Autodesk Inventor part; units mm, degrees
(part 3 of 3)
sketch "Sketch19" plane through (0, 0, -25.4) normal (0, 0, -1) x (-1, 0, 0)
  circle A0 centre (0, 0) radius 236.22 projected
  arc A1 (202.9027, -10.9875) -> (-203.2, 0) centre (0, 0) ccw construction
  circle A2 centre (0, 0) radius 127 construction
  line L0 (127.9212, -89.6882) -> (127.759, -89.2068)
  spline S0 degree 2 poles (127.759, -89.2068) (129.2741, -86.0586) (132.1163, -79.2182) knots 0 0 0 1 1 1
  spline S1 degree 2 poles (132.1163, -79.2182) (135.0319, -72.2013) (136.1206, -69.0829) knots 0 0 0 1 1 1
  line L1 (136.1206, -69.0829) -> (136.5138, -68.884)
  line L2 (136.5138, -68.884) -> (138.7645, -69.8192)
  line L3 (138.7645, -69.8192) -> (138.945, -70.2565)
  spline S2 degree 2 poles (138.945, -70.2565) (137.728, -73.6838) (137.6586, -74.2243) knots 0 0 0 1 1 1
  spline S3 degree 2 poles (137.6586, -74.2243) (137.52, -75.3052) (138.4359, -75.841) knots 0 0 0 1 1 1
  spline S4 degree 2 poles (138.4359, -75.841) (140.5915, -77.2542) (148.4027, -80.4998) knots 0 0 0 1 1 1
  line L4 (148.4027, -80.4998) -> (170.5125, -89.6866)
  line L5 (170.5125, -89.6866) -> (158.5776, -76.1887)
  spline S5 degree 2 poles (158.5776, -76.1887) (157.5986, -75.0575) (151.177, -68.0939) knots 0 0 0 1 1 1
  line L6 (151.177, -68.0939) -> (140.5896, -56.7084)
  line L7 (140.5896, -56.7084) -> (141.5064, -54.5019)
  spline S6 degree 2 poles (141.5064, -54.5019) (146.2817, -54.4678) (153.6703, -54.1223) knots 0 0 0 1 1 1
  line L8 (153.6703, -54.1223) -> (165.2679, -53.6109)
  line L9 (165.2679, -53.6109) -> (186.6543, -52.4575)
  line L10 (186.6543, -52.4575) -> (163.9708, -43.0323)
  spline S7 degree 2 poles (163.9708, -43.0323) (156.1596, -39.7867) (153.6556, -39.212) knots 0 0 0 1 1 1
  spline S8 degree 2 poles (153.6556, -39.212) (152.6113, -38.9851) (151.9615, -39.8019) knots 0 0 0 1 1 1
  spline S9 degree 2 poles (151.9615, -39.8019) (151.6274, -40.2323) (150.0572, -43.5129) knots 0 0 0 1 1 1
  line L11 (150.0572, -43.5129) -> (149.62, -43.6935)
  line L12 (149.62, -43.6935) -> (147.3693, -42.7583)
  line L13 (147.3693, -42.7583) -> (147.2328, -42.3394)
  spline S10 degree 2 poles (147.2328, -42.3394) (148.968, -38.6616) (150.3249, -35.3958) knots 0 0 0 1 1 1
  spline S11 degree 2 poles (150.3249, -35.3958) (151.8836, -31.6447) (153.284, -27.776) knots 0 0 0 1 1 1
  line L14 (153.284, -27.776) -> (153.6772, -27.5771)
  line L15 (153.6772, -27.5771) -> (155.9279, -28.5123)
  line L16 (155.9279, -28.5123) -> (156.1084, -28.9496)
  spline S12 degree 2 poles (156.1084, -28.9496) (154.8913, -32.3769) (154.822, -32.9174) knots 0 0 0 1 1 1
  spline S13 degree 2 poles (154.822, -32.9174) (154.7017, -33.9542) (155.5993, -34.5341) knots 0 0 0 1 1 1
  spline S14 degree 2 poles (155.5993, -34.5341) (157.7549, -35.9473) (165.5661, -39.1929) knots 0 0 0 1 1 1
  line L17 (165.5661, -39.1929) -> (182.8656, -46.381)
  spline S15 degree 2 poles (182.8656, -46.381) (190.6327, -49.6083) (193.1991, -50.1572) knots 0 0 0 1 1 1
  spline S16 degree 2 poles (193.1991, -50.1572) (194.1993, -50.3657) (194.8491, -49.549) knots 0 0 0 1 1 1
  spline S17 degree 2 poles (194.8491, -49.549) (195.1832, -49.1186) (196.7533, -45.8379) knots 0 0 0 1 1 1
  line L18 (196.7533, -45.8379) -> (197.2348, -45.6757)
  line L19 (197.2348, -45.6757) -> (199.4413, -46.5926)
  line L20 (199.4413, -46.5926) -> (199.6219, -47.0298)
  spline S18 degree 2 poles (199.6219, -47.0298) (197.9893, -50.3363) (195.8255, -55.5438) knots 0 0 0 1 1 1
  spline S19 degree 2 poles (195.8255, -55.5438) (194.1569, -59.5597) (193.1489, -62.6082) knots 0 0 0 1 1 1
  spline S20 degree 2 poles (193.1489, -62.6082) (190.2192, -62.6846) (184.8485, -62.7818) knots 0 0 0 1 1 1
  line L21 (184.8485, -62.7818) -> (179.4852, -62.9856)
  line L22 (179.4852, -62.9856) -> (153.401, -64.3605)
  line L23 (153.401, -64.3605) -> (161.4791, -73.5648)
  line L24 (161.4791, -73.5648) -> (174.9592, -88.3257)
  spline S21 degree 2 poles (174.9592, -88.3257) (177.3293, -90.9665) (180.2397, -93.6766) knots 0 0 0 1 1 1
  spline S22 degree 2 poles (180.2397, -93.6766) (178.4788, -97.292) (177.947, -98.5718) knots 0 0 0 1 1 1
  spline S23 degree 2 poles (177.947, -98.5718) (175.2881, -104.9708) (174.0969, -108.4606) knots 0 0 0 1 1 1
  line L25 (174.0969, -108.4606) -> (173.6412, -108.6853)
  line L26 (173.6412, -108.6853) -> (171.3905, -107.7501)
  line L27 (171.3905, -107.7501) -> (171.2283, -107.2687)
  spline S24 degree 2 poles (171.2283, -107.2687) (172.4271, -103.8855) (172.4964, -103.345) knots 0 0 0 1 1 1
  spline S25 degree 2 poles (172.4964, -103.345) (172.635, -102.2641) (171.7816, -101.7025) knots 0 0 0 1 1 1
  spline S26 degree 2 poles (171.7816, -101.7025) (169.5635, -100.3152) (161.7964, -97.0879) knots 0 0 0 1 1 1
  line L28 (161.7964, -97.0879) -> (144.497, -89.8998)
  spline S27 degree 2 poles (144.497, -89.8998) (136.6857, -86.6541) (134.1817, -86.0795) knots 0 0 0 1 1 1
  spline S28 degree 2 poles (134.1817, -86.0795) (133.1375, -85.8526) (132.4693, -86.7134) knots 0 0 0 1 1 1
  spline S29 degree 2 poles (132.4693, -86.7134) (132.1352, -87.1439) (130.5834, -90.3804) knots 0 0 0 1 1 1
  line L29 (130.5834, -90.3804) -> (130.1278, -90.6051)
  line L30 (130.1278, -90.6051) -> (127.9212, -89.6882)
  line L31 (96.1488, -143.05) -> (96.1692, -142.5097)
  spline S30 degree 2 poles (96.1692, -142.5097) (97.389, -140.6622) (96.6476, -138.808) (92.3916, -134.2169) knots 0 0 0 1 2 2 2
  spline S31 degree 2 poles (92.3916, -134.2169) (90.3448, -132.0089) (88.1527, -130.066) knots 0 0 0 1 1 1
  spline S32 degree 2 poles (88.1527, -130.066) (93.7904, -118.7143) (100.8699, -112.1516) knots 0 0 0 1 1 1
  spline S33 degree 2 poles (100.8699, -112.1516) (110.1574, -103.5421) (131.3344, -103.3298) (139.6516, -112.3018) knots 0 0 0 1 2 2 2
  spline S34 degree 2 poles (139.6516, -112.3018) (150.5028, -124.0075) (144.9851, -138.441) knots 0 0 0 1 1 1
  spline S35 degree 2 poles (144.9851, -138.441) (142.4707, -145.0075) (135.286, -151.6677) knots 0 0 0 1 1 1
  spline S36 degree 2 poles (135.286, -151.6677) (131.1505, -155.5014) (126.03, -158.5538) knots 0 0 0 1 1 1
  spline S37 degree 2 poles (126.03, -158.5538) (121.8106, -161.0317) (118.9006, -161.9698) knots 0 0 0 1 1 1
  line L32 (118.9006, -161.9698) -> (118.268, -161.7091)
  spline S38 degree 2 poles (118.268, -161.7091) (116.7896, -158.7787) (111.9795, -152.7463) knots 0 0 0 1 1 1
  line L33 (111.9795, -152.7463) -> (112.035, -152.1735)
  line L34 (112.035, -152.1735) -> (113.5771, -150.744)
  line L35 (113.5771, -150.744) -> (114.0823, -150.7969)
  spline S39 degree 2 poles (114.0823, -150.7969) (114.5372, -151.2876) (117.6065, -154.1768) (118.3665, -154.6452) knots 0 0 0 1 2 2 2
  spline S40 degree 2 poles (118.3665, -154.6452) (120.9175, -155.1476) (124.7259, -153.7025) knots 0 0 0 1 1 1
  spline S41 degree 2 poles (124.7259, -153.7025) (128.7095, -152.095) (132.1441, -148.911) knots 0 0 0 1 1 1
  spline S42 degree 2 poles (132.1441, -148.911) (141.3614, -140.3665) (137.9785, -129.6877) knots 0 0 0 1 1 1
  spline S43 degree 2 poles (137.9785, -129.6877) (136.4068, -124.7586) (132.2157, -120.2375) knots 0 0 0 1 1 1
  spline S44 degree 2 poles (132.2157, -120.2375) (125.523, -113.0178) (117.2819, -111.8602) knots 0 0 0 1 1 1
  spline S45 degree 2 poles (117.2819, -111.8602) (108.7056, -110.6223) (102.292, -116.5678) knots 0 0 0 1 1 1
  spline S46 degree 2 poles (102.292, -116.5678) (98.8924, -119.7192) (97.0352, -124.1126) knots 0 0 0 1 1 1
  spline S47 degree 2 poles (97.0352, -124.1126) (98.5494, -126.0975) (101.5058, -129.2868) knots 0 0 0 1 1 1
  spline S48 degree 2 poles (101.5058, -129.2868) (103.8775, -131.8452) (104.5726, -132.2435) knots 0 0 0 1 1 1
  spline S49 degree 2 poles (104.5726, -132.2435) (105.1052, -132.4666) (106.1062, -131.9296) knots 0 0 0 1 1 1
  spline S50 degree 2 poles (106.1062, -131.9296) (106.9371, -131.42) (110.8795, -128.2215) knots 0 0 0 1 1 1
  line L36 (110.8795, -128.2215) -> (111.3873, -128.207)
  line L37 (111.3873, -128.207) -> (112.9143, -129.8542)
  line L38 (112.9143, -129.8542) -> (112.8613, -130.3594)
  spline S51 degree 2 poles (112.8613, -130.3594) (108.9788, -133.7631) (104.8757, -137.6318) knots 0 0 0 1 1 1
  spline S52 degree 2 poles (104.8757, -137.6318) (102.525, -139.8761) (97.8262, -144.2971) knots 0 0 0 1 1 1
  line L39 (97.8262, -144.2971) -> (97.3184, -144.3117)
  line L40 (97.3184, -144.3117) -> (96.1488, -143.05)
  line L41 (26.9755, -152.7156) -> (27.1725, -152.2854)
  spline S53 degree 2 poles (27.1725, -152.2854) (30.5538, -151.2323) (37.4968, -148.651) knots 0 0 0 1 1 1
  spline S54 degree 2 poles (37.4968, -148.651) (44.5743, -146.0198) (47.6432, -144.6749) knots 0 0 0 1 1 1
  line L42 (47.6432, -144.6749) -> (48.0567, -144.8271)
  line L43 (48.0567, -144.8271) -> (48.906, -147.1115)
  line L44 (48.906, -147.1115) -> (48.6642, -147.5583)
  spline S55 degree 2 poles (48.6642, -147.5583) (45.3713, -148.9865) (44.8837, -149.3207) knots 0 0 0 1 1 1
  spline S56 degree 2 poles (44.8837, -149.3207) (44.043, -149.9392) (44.2302, -150.9913) knots 0 0 0 1 1 1
  spline S57 degree 2 poles (44.2302, -150.9913) (44.7097, -153.5152) (47.6573, -161.4437) knots 0 0 0 1 1 1
  line L45 (47.6573, -161.4437) -> (50.6216, -169.417)
  spline S58 degree 2 poles (50.6216, -169.417) (52.3456, -168.98) (61.4387, -165.5994) knots 0 0 0 1 1 1
  spline S59 degree 2 poles (61.4387, -165.5994) (69.8152, -162.4852) (72.3914, -161.3235) knots 0 0 0 1 1 1
  line L46 (72.3914, -161.3235) -> (69.4271, -153.3502)
  spline S60 degree 2 poles (69.4271, -153.3502) (66.4794, -145.4217) (65.1489, -143.2142) knots 0 0 0 1 1 1
  spline S61 degree 2 poles (65.1489, -143.2142) (64.6481, -142.2787) (63.5627, -142.3763) knots 0 0 0 1 1 1
  spline S62 degree 2 poles (63.5627, -142.3763) (63.02, -142.4251) (59.5491, -143.5116) knots 0 0 0 1 1 1
  line L47 (59.5491, -143.5116) -> (59.119, -143.3146)
  line L48 (59.119, -143.3146) -> (58.2863, -141.0749)
  line L49 (58.2863, -141.0749) -> (58.4833, -140.6448)
  spline S63 degree 2 poles (58.4833, -140.6448) (61.8646, -139.5916) (68.7629, -137.027) knots 0 0 0 1 1 1
  spline S64 degree 2 poles (68.7629, -137.027) (75.8851, -134.3791) (78.9093, -133.0508) knots 0 0 0 1 1 1
  line L50 (78.9093, -133.0508) -> (79.3675, -133.1864)
  line L51 (79.3675, -133.1864) -> (80.2168, -135.4709)
  line L52 (80.2168, -135.4709) -> (79.9751, -135.9176)
  spline S65 degree 2 poles (79.9751, -135.9176) (76.6821, -137.3458) (76.1946, -137.68) knots 0 0 0 1 1 1
  spline S66 degree 2 poles (76.1946, -137.68) (75.3538, -138.2985) (75.541, -139.3506) knots 0 0 0 1 1 1
  spline S67 degree 2 poles (75.541, -139.3506) (76.0205, -141.8746) (78.9682, -149.8031) knots 0 0 0 1 1 1
  line L53 (78.9682, -149.8031) -> (85.4963, -167.3622)
  spline S68 degree 2 poles (85.4963, -167.3622) (88.4272, -175.2459) (89.7297, -177.5149) knots 0 0 0 1 1 1
  spline S69 degree 2 poles (89.7297, -177.5149) (90.2586, -178.3889) (91.2992, -178.308) knots 0 0 0 1 1 1
  spline S70 degree 2 poles (91.2992, -178.308) (91.8866, -178.2425) (95.3128, -177.1727) knots 0 0 0 1 1 1
  line L54 (95.3128, -177.1727) -> (95.8044, -177.3978)
  line L55 (95.8044, -177.3978) -> (96.637, -179.6375)
  line L56 (96.637, -179.6375) -> (96.3952, -180.0843)
  spline S71 degree 2 poles (96.3952, -180.0843) (93.1316, -181.0427) (86.099, -183.6573) knots 0 0 0 1 1 1
  spline S72 degree 2 poles (86.099, -183.6573) (78.8872, -186.3385) (75.9693, -187.6782) knots 0 0 0 1 1 1
  line L57 (75.9693, -187.6782) -> (75.5392, -187.4812)
  line L58 (75.5392, -187.4812) -> (74.6898, -185.1968)
  line L59 (74.6898, -185.1968) -> (74.8868, -184.7666)
  spline S73 degree 2 poles (74.8868, -184.7666) (78.2245, -183.3218) (78.6673, -183.0042) knots 0 0 0 1 1 1
  spline S74 degree 2 poles (78.6673, -183.0042) (79.5529, -182.3691) (79.3375, -181.3785) knots 0 0 0 1 1 1
  spline S75 degree 2 poles (79.3375, -181.3785) (78.8862, -178.7931) (75.9552, -170.9094) knots 0 0 0 1 1 1
  line L60 (75.9552, -170.9094) -> (73.9068, -165.3997)
  spline S76 degree 2 poles (73.9068, -165.3997) (70.3182, -166.581) (64.1366, -168.8791) knots 0 0 0 1 1 1
  spline S77 degree 2 poles (64.1366, -168.8791) (54.4612, -172.4762) (52.1371, -173.4932) knots 0 0 0 1 1 1
  line L61 (52.1371, -173.4932) -> (54.1854, -179.0029)
  spline S78 degree 2 poles (54.1854, -179.0029) (57.1164, -186.8866) (58.4188, -189.1556) knots 0 0 0 1 1 1
  spline S79 degree 2 poles (58.4188, -189.1556) (58.9477, -190.0296) (59.9883, -189.9487) knots 0 0 0 1 1 1
  spline S80 degree 2 poles (59.9883, -189.9487) (60.5758, -189.8832) (64.0019, -188.8134) knots 0 0 0 1 1 1
  line L62 (64.0019, -188.8134) -> (64.4935, -189.0385)
  line L63 (64.4935, -189.0385) -> (65.3262, -191.2782)
  line L64 (65.3262, -191.2782) -> (65.1292, -191.7083)
  spline S81 degree 2 poles (65.1292, -191.7083) (61.8208, -192.6834) (54.833, -195.2813) knots 0 0 0 1 1 1
  spline S82 degree 2 poles (54.833, -195.2813) (47.5764, -197.9792) (44.6584, -199.3189) knots 0 0 0 1 1 1
  line L65 (44.6584, -199.3189) -> (44.2283, -199.1219)
  line L66 (44.2283, -199.1219) -> (43.379, -196.8374)
  line L67 (43.379, -196.8374) -> (43.576, -196.4073)
  spline S83 degree 2 poles (43.576, -196.4073) (46.9585, -194.9458) (47.3565, -194.6449) knots 0 0 0 1 1 1
  spline S84 degree 2 poles (47.3565, -194.6449) (48.242, -194.0098) (48.0267, -193.0191) knots 0 0 0 1 1 1
  spline S85 degree 2 poles (48.0267, -193.0191) (47.5753, -190.4337) (44.6443, -182.55) knots 0 0 0 1 1 1
  line L68 (44.6443, -182.55) -> (38.1162, -164.9909)
  spline S86 degree 2 poles (38.1162, -164.9909) (35.1686, -157.0624) (33.838, -154.8549) knots 0 0 0 1 1 1
  spline S87 degree 2 poles (33.838, -154.8549) (33.3373, -153.9194) (32.2519, -154.017) knots 0 0 0 1 1 1
  spline S88 degree 2 poles (32.2519, -154.017) (31.7092, -154.0658) (28.2383, -155.1522) knots 0 0 0 1 1 1
  line L69 (28.2383, -155.1522) -> (27.8081, -154.9553)
  line L70 (27.8081, -154.9553) -> (26.9755, -152.7156)
  dimension "d113" = 406.4
  dimension "d117" = 254
  constraints: 2 centre point, 2 coincident, 2 point on circle, 1 other
  measures "d113" diameter of A1
  measures "d117" diameter of A2
emboss "Emboss2" sketch "Sketch19" operation add depth 3.175 direction (0, 0, 1) contours L0 S0 S1 L1 L2 L3 S2 S3 S4 L4 L5 S5 L6 L7 S6 L8 L9 L10 S7 S8 S9 L11 L12 L13 S10 S11 L14 L15 L16 S12 S13 S14 L17 S15 S16 S17 L18 L19 L20 S18 S19 S20 L21 L22 L23 L24 S21 S22 S23 L25 L26 L27 S24 S25 S26 L28 S27 S28 S29 L29 L30 | L31 S30 S31 S32 S33 S34 S35 S36 S37 L32 S38 L33 L34 L35 S39 S40 S41 S42 S43 S44 S45 S46 S47 S48 S49 S50 L36 L37 L38 S51 S52 L39 L40 | L41 S53 S54 L42 L43 L44 S55 S56 S57 L45 S58 S59 L46 S60 S61 S62 L47 L48 L49 S63 S64 L50 L51 L52 S65 S66 S67 L53 S68 S69 S70 L54 L55 L56 S71 S72 L57 L58 L59 S73 S74 S75 L60 S76 S77 L61 S78 S79 S80 L62 L63 L64 S81 S82 L65 L66 L67 S83 S84 S85 L68 S86 S87 S88 L69 L70
sketch "Sketch25" plane through (0, 0, 0) normal (0, 0, 1) x (1, 0, 0)
  line L0 (-238.508, 0) -> (258.7625, 0)
  line L1 (258.7625, 0) -> (258.7625, 247.65)
  line L2 (258.7625, 247.65) -> (-238.508, 247.65)
  line L3 (-238.508, 247.65) -> (-238.508, 0)
  point P0 (0, 0)
  constraints: 8 end point, 2 parallel, 1 horizontal, 1 perpendicular
extrude "Extrusion19" cut sketch "Sketch25" against normal through all bodies 2
sketch "Sketch27" plane through (0, 0, -25.4) normal (0, 0, -1) x (-1, 0, 0)
  line L0 (63.5, 0) -> (236.22, 0) projected
  line L1 (223.52, 0) -> (160.02, 0)
  line L2 (160.02, 0) -> (160.02, -19.05)
  line L3 (160.02, -19.05) -> (223.52, -19.05)
  line L4 (223.52, -19.05) -> (223.52, 0)
  arc A0 (-98.1276, -19.05) -> (98.1276, -19.05) centre (0, 0) ccw projected
  line L5 (127, -19.05) -> (98.1276, -19.05) projected
  line L6 (-98.1276, -19.05) -> (-127, -19.05) projected
  line L7 (127, 0) -> (127, -19.05) projected
  line L8 (-127, -19.05) -> (-127, 0) projected
  arc A1 (-98.1276, -19.05) -> (98.1276, -19.05) centre (0, 0) ccw projected
  line L9 (0, -99.9596) -> (0, 0)
  line L10 (-223.52, 0) -> (-160.02, 0)
  line L11 (-160.02, 0) -> (-160.02, -19.05)
  line L12 (-160.02, -19.05) -> (-223.52, -19.05)
  line L13 (-223.52, -19.05) -> (-223.52, 0)
  dimension "d140" = 19.05
  dimension "d141" = 19.05
  dimension "d142" = 63.5
  dimension "d143" = 12.7
  constraints: 18 end point, 4 symmetric about line, 2 parallel, 2 point on circle, 1 horizontal, 1 perpendicular, 1 point on line, 1 vertical
  measures "d140" distance between parallel lines of L0 L5
  measures "d141" distance of L1.end L2.end
  measures "d142" distance of L2.end L3.end
  measures "d143" distance from line of L0.end L4
extrude "Extrusion20" add sketch "Sketch27" along normal blind 25.4 bodies 2
sketch "Sketch28" plane through (-223.52, -19.05, -25.4) normal (0, -1, 0) x (1, 0, 0)
  circle A0 centre (431.8, -12.7) radius 3.3782
  circle A1 centre (398.78, -12.7) radius 3.3782
  line L0 (447.04, 0) -> (447.04, -25.4) projected
  line L1 (383.54, 0) -> (383.54, -25.4) projected
  line L2 (447.04, -25.4) -> (383.54, -25.4) projected
  line L3 (321.6476, 50.8) -> (125.3924, 50.8) projected
  line L4 (223.52, 50.8) -> (223.52, -50.8)
  circle A2 centre (15.24, -12.7) radius 3.3782
  circle A3 centre (48.26, -12.7) radius 3.3782
  line L5 (0, 0) -> (0, -25.4)
  line L6 (63.5, 0) -> (63.5, -25.4)
  line L7 (0, -25.4) -> (63.5, -25.4)
  point P0 (223.52, 25.4)
  dimension "d146" = 6.7564
  dimension "d147" = 6.7564
  dimension "d148" = 15.24
  dimension "d149" = 15.24
  dimension "d150" = 12.7
  dimension "d151" = 25.4
  dimension "d152" = 12.7
  constraints: 8 end point, 6 symmetric about line, 4 centre point, 1 midpoint, 1 vertical, 2 other
  measures "d146" diameter of A0
  measures "d147" diameter of A1
  measures "d148" distance from line of L0 A0.centre
  measures "d149" distance from line of L1 A1.centre
  measures "d150" distance from line of L2 A1.centre
  measures "d151" distance of L1.start L1.end
  measures "d152" distance from line of L2 A0.centre
extrude "Extrusion21" cut sketch "Sketch28" against normal through all bodies 2
sketch "Sketch29" plane through (0, 0, -25.4) normal (0, 0, -1) x (-1, 0, 0)
  line L0 (0, 0) -> (0, -404.1913)
  line L1 (10.16, -139.7) -> (-10.16, -139.7)
  line L2 (63.5, -63.5) -> (-63.5, -63.5) projected
  arc A0 (-236.22, 0) -> (236.22, 0) centre (0, 0) ccw projected
  arc A1 (-10.16, -236.0014) -> (10.16, -236.0014) centre (0, 0) ccw
  line L3 (10.16, -236.0014) -> (10.16, -139.7)
  line L4 (-10.16, -139.7) -> (-10.16, -236.0014)
  dimension "d158" = 76.2
  dimension "d162" = 20.32
  dimension "d163" = 10.16
  dimension "d164" = 10.16
  constraints: 8 end point, 4 point on circle, 2 vertical, 1 centre point, 1 coincident, 1 horizontal, 1 parallel
  measures "d158" distance between parallel lines of L2 L1
  measures "d162" distance between parallel lines of L4 L3
  measures "d163" distance between parallel lines of L4 L0
  measures "d164" distance between parallel lines of L0 L3
extrude "Extrusion22" add sketch "Sketch29" along normal blind 20.32 bodies 2
sketch "Sketch32" plane through (0, 0, 0) normal (0, 0, 1) x (1, 0, 0)
  line L0 (10.16, -236.0014) -> (10.16, -139.7) projected
  line L1 (-10.16, -139.7) -> (-10.16, -236.0014) projected
  line L2 (10.16, -139.7) -> (-10.16, -139.7) projected
  arc A0 (-10.16, -236.0014) -> (10.16, -236.0014) centre (0, 0) ccw
  point P0 (0, 0)
  constraints: 2 point on circle, 1 centre point
extrude "Extrusion23" add sketch "Sketch32" along normal blind 20.32 bodies 2
sketch "Sketch33" plane through (-10.16, -236.0014, -25.4) normal (-1, 0, 0) x (0, 0, 1)
  circle A0 centre (-10.16, 24.0754) radius 3.3782
  circle A1 centre (-10.16, 48.1507) radius 3.3782
  circle A2 centre (-10.16, 72.2261) radius 3.3782
  line L0 (-20.32, 0) -> (-20.32, 96.3014) projected
  line L1 (0, 0) -> (0, 236.0014) projected
  line L2 (0, 96.3014) -> (-20.32, 96.3014) projected
  line L3 (0, 0) -> (-20.32, 0) projected
  circle A3 centre (35.56, 24.0754) radius 3.3782
  circle A4 centre (35.56, 48.1507) radius 3.3782
  circle A5 centre (35.56, 72.2261) radius 3.3782
  line L4 (45.72, 96.3014) -> (45.72, 0) projected
  point P0 (25.4, 236.0014)
  dimension "d167" = 6.7564
  dimension "d168" = 6.7564
  dimension "d169" = 6.7564
  dimension "d170" = 20.32
  dimension "d171" = 10.16
  dimension "d172" = 0
  dimension "d173" = 0
  dimension "d174" = 24.0754
  dimension "d175" = 96.3014
  dimension "d176" = 24.0754
  dimension "d177" = 24.0754
  dimension "d178" = 6.7564
  dimension "d179" = 6.7564
  dimension "d180" = 6.7564
  dimension "d181" = 0
  dimension "d182" = 0
  dimension "d183" = 24.0754
  dimension "d184" = 24.0754
  dimension "d187" = 10.16
  constraints: 6 centre point
  measures "d167" diameter of A0
  measures "d168" diameter of A1
  measures "d169" diameter of A2
  measures "d170" distance between parallel lines of L0 L1
  measures "d171" distance from line of L0 A0.centre
  measures "d172" horizontal distance of A0.centre A1.centre
  measures "d173" horizontal distance of A2.centre A1.centre
  measures "d174" distance from line of L2 A2.centre
  measures "d175" distance between parallel lines of L2 L3
  measures "d176" distance of A2.centre A1.centre
  measures "d177" distance of A1.centre A0.centre
  measures "d178" diameter of A3
  measures "d179" diameter of A4
  measures "d180" diameter of A5
  measures "d181" horizontal distance of A3.centre A4.centre
  measures "d182" horizontal distance of A5.centre A4.centre
  measures "d183" distance of A5.centre A4.centre
  measures "d184" distance of A4.centre A3.centre
  measures "d187" distance from line of L4 A3.centre
extrude "Extrusion24" cut sketch "Sketch33" against normal through all contours A0 | A1 | A2 | A3 | A4 | A5 bodies 2
sketch "Sketch35" plane through (0, 0, 25.4) normal (0, 0, 1) x (1, 0, 0)
  line L0 (45, -104.14) -> (-45, -104.14)
  line L1 (45, -104.14) -> (45, -89.2577)
  arc A0 (-98.1276, -19.05) -> (98.1276, -19.05) centre (0, 0) ccw projected
  line L2 (-45, -104.14) -> (-45, -89.2577)
  arc A1 (-45, -89.2577) -> (45, -89.2577) centre (0, 0) ccw
  dimension "d195" = 104.14
  dimension "d196" = 90
  constraints: 6 end point, 4 point on circle, 1 centre point, 1 coincident, 1 horizontal, 1 parallel, 1 vertical
  measures "d195" distance from line of point (0, 0) L0
  measures "d196" distance of L0.start L0.end
extrude "Extrusion26" add sketch "Sketch35" against normal up to surface (25.4 mm away) bodies 1
sketch "Sketch36" plane through (-45, -104.14, 25.4) normal (0, -1, 0) x (1, 0, 0)
  circle A0 centre (76.5, -12.7) radius 4
  circle A1 centre (13.5, -12.7) radius 4
  line L0 (90, 0) -> (90, -25.4) projected
  line L1 (0, 0) -> (90, 0) projected
  line L2 (0, 0) -> (0, -25.4) projected
  point P0 (45, -25.4)
  dimension "d200" = 63
  dimension "d201" = 8
  dimension "d202" = 8
  dimension "d203" = 13.5
  dimension "d204" = 12.7
  dimension "d205" = 13.5
  dimension "d206" = 12.7
  constraints: 2 centre point
  measures "d200" distance of A1.centre A0.centre
  measures "d201" diameter of A0
  measures "d202" diameter of A1
  measures "d203" distance from line of A0.centre L0
  measures "d204" distance from line of L1 A0.centre
  measures "d205" distance from line of L2 A1.centre
  measures "d206" distance from line of L1 A1.centre
extrude "Extrusion27" cut sketch "Sketch36" against normal blind 10 bodies 1
sketch "Sketch38" plane through (0, 0, 25.4) normal (0, 0, 1) x (1, 0, 0)
  line L0 (0, 0) -> (285.75, 0)
  line L1 (285.75, 0) -> (285.75, -287.3375)
  line L2 (285.75, -287.3375) -> (0, -287.3375)
  line L3 (0, -287.3375) -> (0, 0)
  constraints: 8 end point, 2 parallel, 1 horizontal, 1 perpendicular
extrude "Extrusion28" cut sketch "Sketch38" along normal mid plane 200 bodies 1
sketch "Sketch39" plane through (0, 0, -25.4) normal (0, 0, -1) x (-1, 0, 0)
  line L0 (0, 0) -> (-358.775, 0)
  line L1 (-358.775, 0) -> (-358.775, -306.3875)
  line L2 (-358.775, -306.3875) -> (0, -306.3875)
  line L3 (0, -306.3875) -> (0, 0)
  constraints: 8 end point, 2 parallel, 1 horizontal, 1 perpendicular
extrude "Extrusion29" cut sketch "Sketch39" along normal mid plane 200 bodies 2
equation "\"d36\" = 0.25 * d33"
equation "\"d39\" = 0.25 * d33"
equation "\"d41\" = d40"
equation "\"d37\" = d36"
body "Solid1"
body "Solid3"
